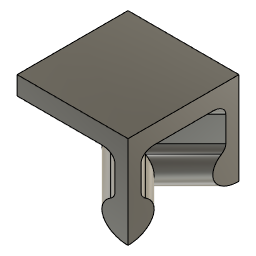
_Tooth Prototype.e5bad83f-fe98-483c-a222-4c0f021ca759 (Autodesk Fusion 360 design; units mm, degrees)
Autodesk Fusion 360 part; units mm, degrees
sketch "Sketch1" plane through (0, 0, 0) normal (0, 0, 1) x (1, 0, 0)
  line L0 (-15, -15) -> (15, -15)
  line L1 (15, -15) -> (15, 15)
  line L2 (15, 15) -> (-15, 15)
  line L3 (-15, 15) -> (-15, -15)
  line L4 (-15, -15) -> (15, 15) construction
  line L5 (15, -15) -> (-15, 15) construction
  line L6 (-25, 25) -> (25, 25)
  line L7 (25, 25) -> (25, -25)
  line L8 (25, -25) -> (-25, -25)
  line L9 (-25, -25) -> (-25, 25)
  line L10 (15, -15) -> (25, -25) construction
  line L11 (-25, 25) -> (-15, 15) construction
  line L12 (15, 15) -> (25, 25) construction
  line L13 (-15, -15) -> (-25, -25) construction
  dimension "d1" = 30
  dimension "d2" = 30
  dimension "d23" = 10
  dimension "d24" = 10
  dimension "d25" = 10
  dimension "d26" = 10
  constraint horizontal L0
  constraint vertical L1
  constraint horizontal L2
  constraint vertical L3
  constraint coincident origin L4
  constraint coincident origin L5
  constraint horizontal L6
  constraint vertical L7
  constraint horizontal L8
  constraint vertical L9
  measures "d1" distance of L0 L2
  measures "d2" distance of L1 L3
  measures "d23" distance of L1 L7
  measures "d24" distance of L2 L6
  measures "d25" distance of L3 L9
  measures "d26" distance of L0 L8
extrude "Extrude1" add sketch "Sketch1" along normal blind 5 contours L0 L1 L2 L3
ref_plane "WorkPlane1" through (0, 0, 0) normal (0.707107, 0.707107, 0) x (-0.707107, 0.707107, 0)
ref_plane "WorkPlane2" through (0, 0, 0) normal (0.707107, -0.707107, 0) x (0.707107, 0.707107, 0)
sketch "Sketch2" plane through (0, 0, 0) normal (0.707107, 0.707107, 0) x (-0.707107, 0.707107, 0)
  circle A0 centre (0, -15) radius 5
  line L0 (2.5, -10.6699) -> (2.5, -2.5)
  line L1 (-2.5, -10.6699) -> (-2.5, -2.5)
  arc A1 (5, 0) -> (2.5, -2.5) centre (5, -2.5) ccw
  arc A2 (-2.5, -2.5) -> (-5, 0) centre (-5, -2.5) ccw
  line L2 (0, 0) -> (0, -15) construction
  line L3 (0, -7.5) -> (2.5, -7.5) construction
  line L4 (0, -7.5) -> (-2.5, -7.5) construction
  line L5 (21.2132, 0) -> (0, 0)
  line L6 (0, 0) -> (-21.2132, 0)
  line L7 (5, -2.5) -> (-5, -2.5) construction
  arc A3 (2.5, -9.4098) -> (3.3333, -11.2732) centre (5, -9.4098) ccw
  arc A4 (-3.3333, -11.2732) -> (-2.5, -9.4098) centre (-5, -9.4098) ccw
  line L8 (-17.2446, 0) -> (-17.2446, -26.2222)
  line L9 (-17.2446, -26.2222) -> (15.3661, -26.2222)
  line L10 (15.3661, -26.2222) -> (15.3661, 0)
  line L11 (0, -20) -> (0, -26.2222)
  dimension "d7" = 10
  dimension "d8" = 5
  dimension "d9" = 15
  dimension "d14" = 2.5
  constraint coincident A0 L0.start
  constraint vertical L0
  constraint coincident A0 L1.start
  constraint parallel L0 L1
  constraint tangent L0 A1
  constraint tangent L1 A2
  constraint coincident L2.start L5.end
  constraint coincident A0.centre L2.end
  constraint vertical L2
  constraint midpoint L2 L3.start
  constraint coincident L0 L3.end
  constraint perpendicular L0 L3
  constraint coincident L1 L4.end
  constraint perpendicular L1 L4
  constraint equal L3 L4
  constraint tangent A2 L6
  constraint tangent A1 L5
  constraint coincident A1.centre L7.start
  constraint coincident A2.centre L7.end
  constraint horizontal L7
  constraint coincident A1.start L5
  constraint coincident A2.end L6
  constraint tangent A0 A4
  constraint tangent L1 A4
  constraint tangent L0 A3
  constraint tangent A0 A3
  constraint equal A3 A4
  constraint coincident L0 A3.start
  constraint coincident A0 A3.end
  constraint coincident A0 A4.start
  constraint coincident L1 A4.end
  constraint equal A1 A3
  constraint coincident L6 L8.start
  constraint perpendicular L6 L8
  constraint coincident L5 L10.end
  constraint horizontal L9
  constraint vertical L10
  constraint coincident A0 L11.start
  constraint coincident L9 L11.end
  constraint perpendicular L9 L11
  measures "d7" diameter of A0
  measures "d8" distance of L3.end L4.end
  measures "d9" distance of L2.start A0.centre
  measures "d14" radius of A1
extrude "Extrude2" add sketch "Sketch2" along normal blind 25 and the other way blind 5 contours A0 | A0 L0 A3 | A0 L0 L1 A1 A2 L5 L6 | A0 L1 A4
sketch "Sketch3" plane through (0, 0, 0) normal (0.707107, -0.707107, 0) x (0.707107, 0.707107, 0)
  circle A0 centre (0, -15) radius 5
  line L0 (0, 0) -> (0, -15) construction
  line L1 (-2.5, -2.5) -> (-2.5, -9.4098)
  line L2 (2.5, -2.5) -> (2.5, -9.4098)
  line L3 (-21.2132, 0) -> (0, 0)
  line L4 (0, -5.6591) -> (2.5, -5.6591) construction
  line L5 (0, -5.6591) -> (-2.5, -5.6591) construction
  arc A1 (-3.3333, -11.2732) -> (-2.5, -9.4098) centre (-5, -9.4098) ccw
  arc A2 (2.5, -9.4098) -> (3.3333, -11.2732) centre (5, -9.4098) ccw
  arc A3 (-2.5, -2.5) -> (-5, 0) centre (-5, -2.5) ccw
  line L6 (0, 0) -> (16.2132, 0)
  arc A4 (5, 0) -> (2.5, -2.5) centre (5, -2.5) ccw
  line L7 (-15.7318, 0) -> (-15.7318, -22.3804)
  line L8 (-15.7318, -22.3804) -> (13.46, -22.3804)
  line L9 (13.46, -22.3804) -> (13.46, 0)
  line L10 (0, -20) -> (0, -22.3804)
  line L11 (0, 0) -> (0, -26.2222)
  dimension "d12" = 15
  dimension "d13" = 10
  dimension "d15" = 5
  dimension "d16" = 2.5
  constraint coincident L0.start L3.end
  constraint coincident A0.centre L0.end
  constraint vertical L0
  constraint vertical L1
  constraint parallel L0 L2
  constraint coincident L0 L4.start
  constraint coincident L2 L4.end
  constraint perpendicular L2 L4
  constraint coincident L1 L5.end
  constraint perpendicular L1 L5
  constraint equal L4 L5
  constraint coincident A0 A1.start
  constraint tangent L1 A1
  constraint coincident A0 A2.end
  constraint tangent L2 A2
  constraint coincident L3 A3.end
  constraint tangent L1 A3
  constraint tangent L3 A3
  constraint equal A1 A3
  constraint equal A2 A3
  constraint tangent A0 A1
  constraint tangent A0 A2
  constraint tangent L2 A4
  constraint equal A3 A4
  constraint tangent L6 A4
  constraint coincident L6 A4.start
  constraint coincident L3 L7.start
  constraint perpendicular L3 L7
  constraint perpendicular L7 L8
  constraint coincident L6 L9.end
  constraint perpendicular L6 L9
  constraint coincident A0 L10.start
  constraint coincident L8 L10.end
  constraint perpendicular L8 L10
  constraint collinear L10 L11
  measures "d12" distance of L0.start A0.centre
  measures "d13" diameter of A0
  measures "d15" distance of L4.end L5.end
  measures "d16" radius of A3
extrude "Extrude3" add sketch "Sketch3" along normal blind 25 and the other way blind 5 contours A0 L11 | A0 L2 A2 L6 A4 L11 | A0 L11 | A0 L1 L3 A1 A3 L11
extrude "Extrude4" cut sketch "Sketch1" against normal blind 20
extrude "Extrude5" cut sketch "Sketch2" along normal mid plane 30 contours A0 L0 A1 L5 A3 L9 L10 L11
extrude "Extrude6" cut sketch "Sketch3" along normal mid plane 30 contours A0 L1 L3 A1 A3 L7 L8 L10 L11
equation "d23 = d26"
equation "d24 = d26"
equation "d25 = d26"
